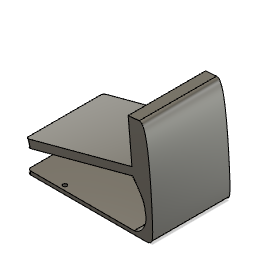
Iron_ Board Clip V2 (Autodesk Fusion 360 design; units mm, degrees)
Autodesk Fusion 360 part; units mm, degrees
sketch "Pi Plate" plane through (0, 0, 0) normal (0, 1, 0) x (1, 0, 0)
  line L0 (0, 0) -> (0, -56)
  line L1 (0, 0) -> (85, 0)
  line L2 (85, 0) -> (85, -56)
  line L3 (85, -56) -> (0, -56)
  line L4 (81.5, 0) -> (81.5, -3.5) construction
  line L5 (81.5, -3.5) -> (85, -3.5) construction
  circle A0 centre (81.5, -3.5) radius 1.425
  line L6 (0, -28) -> (85, -28) construction
  circle A1 centre (81.5, -52.5) radius 1.425
  line L7 (81.5, -3.5) -> (23.5, -3.5) construction
  circle A2 centre (23.5, -3.5) radius 1.425
  circle A3 centre (23.5, -52.5) radius 1.425
  line L8 (85, 0) -> (85, -15)
  line L9 (85, -15) -> (93, -15)
  line L10 (93, -15) -> (93, -5)
  line L11 (93, -5) -> (85, -5)
  dimension "d1" = 56
  dimension "d2" = 85
  dimension "d3" = 3.5
  dimension "d4" = 3.5
  dimension "d6" = 2.85
  dimension "d7" = 58
  dimension "d8" = 2.85
  dimension "d37" = 15
  dimension "d38" = 8
  dimension "d39" = 10
  constraint coincident L0.start L1.start
  constraint vertical L0
  constraint perpendicular L0 L1
  constraint perpendicular L1 L2
  constraint perpendicular L2 L3
  constraint coincident L1 L4.start
  constraint perpendicular L1 L4
  constraint coincident L2 L5.end
  constraint perpendicular L2 L5
  constraint coincident L4.end L5.start
  constraint midpoint L0 L6.start
  constraint midpoint L2 L6.end
  constraint symmetric A0 L6 A1
  constraint perpendicular L4 L7
  constraint coincident L7.end A2.centre
  constraint symmetric L6 A2 A3
  constraint perpendicular L5 L8
  constraint perpendicular L8 L9
  constraint perpendicular L9 L10
  constraint coincident L2 L11.end
  measures "d1" distance of L0.start L0.end
  measures "d2" distance of L0.start L1.end
  measures "d3" distance of L4.start L4.end
  measures "d4" distance of L4.end L5.end
  measures "d6" diameter of A0
  measures "d7" distance of L4.end L7.end
  measures "d8" diameter of A2
  measures "d37" distance of L1.end L8.end
  measures "d38" distance of L8.end L9.end
  measures "d39" distance of L9.end L10.end
extrude "Extrude1" add sketch "Pi Plate" along normal blind 2.5 contours L0 L1 L2 L3 L8
sketch "Clip Side" plane through (0, 0, 56) normal (0, 0, 1) x (1, 0, 0)
  line L0 (0, 0) -> (85, 0)
  line L1 (85, 0) -> (85, 2.5)
  line L2 (85, 2.5) -> (0, 2.5)
  line L3 (0, 2.5) -> (0, 0)
  line L4 (85, 2.5) -> (75.9413, 36.3074) construction
  line L5 (85, 2.5) -> (90, 2.5153)
  line L6 (0, 2.5) -> (0, 15.959)
  line L7 (0, 15.959) -> (75.9413, 36.3074)
  line L8 (74.5178, 41.62) -> (-1.4235, 21.2716)
  line L9 (-1.4235, 21.2716) -> (0, 15.959)
  line L10 (80.4707, 19.4037) -> (138.9269, 35.067) construction
  line L11 (75.9413, 36.3074) -> (84.1517, 38.5074)
  line L12 (72.7687, 72.5706) -> (80.7383, 73.2679)
  line L13 (80.7383, 73.2679) -> (84.1517, 38.5074)
  spline S0 degree 5 poles (85, 0) (85.7038, -0.0126) (86.9919, 0.0407) (88.5662, 0.3597) (89.9346, 1.2401) (90.5461, 4.0966) (90.5133, 11.1599) (90.0253, 22.2132) (89.1744, 36.0508) (87.9366, 50.5661) (86.2276, 63.3649) (84.3878, 70.3523) (82.6924, 72.9385) (81.4143, 73.373) (80.7383, 73.2679) knots 0 0 0 0 0 0 0.1 0.2 0.3 0.4 0.5 0.6 0.7 0.8 0.9 1 1 1 1 1 1
  line L14 (82.5373, 73.5477) -> (78.9392, 72.988)
  line L15 (89.2071, -0.1554) -> (90.7928, 5.1861)
  line L16 (75.9413, 36.3074) -> (72.7687, 72.5706)
  line L17 (74.5178, 41.62) -> (75.9413, 36.3074)
  spline S1 degree 5 poles (77.0666, 2.5) (77.518, 2.582) (78.4018, 2.8013) (79.6705, 3.2963) (81.246, 4.2904) (82.9988, 6.0816) (84.4519, 8.3641) (85.4854, 11.012) (85.8037, 13.7661) (85.5761, 16.347) (85.1435, 18.5645) (84.827, 20.3572) (84.5732, 21.9602) (83.9831, 23.7933) (82.9151, 26.0418) (81.2588, 28.8315) (79.4414, 31.5279) (77.799, 33.8154) (76.5811, 35.4573) (75.9413, 36.3074) knots 0 0 0 0 0 0 0.066667 0.133333 0.2 0.266667 0.333333 0.4 0.466667 0.533333 0.6 0.666667 0.733333 0.8 0.866667 0.933333 1 1 1 1 1 1
  line L18 (85.1921, 18.349) -> (84.3983, 22.7759)
  line L19 (74.5178, 41.62) -> (75.4546, 41.871)
  line L20 (74.355, 54.439) -> (84.8151, 55.3541) construction
  line L21 (83.6776, 68.3559) -> (85.9526, 42.3523) construction
  line L22 (83.6443, 6.1062) -> (86.3557, 13.8938)
  point P0 (84.7952, 20.5625)
  point P1 (85, 10)
  dimension "d12" = 35
  dimension "d13" = 5
  dimension "d15" = 5.5
  dimension "d16" = 31
  dimension "d18" = 8.5
  dimension "d36" = 75
  dimension "d50" = 10.5
  dimension "d51" = 8
  dimension "d52" = 14.8786
  dimension "d53" = 80
  constraint coincident L1.end L2.start
  constraint perpendicular L2 L6
  constraint perpendicular L4 L7
  constraint perpendicular L7 L9
  constraint midpoint L4 L10.start
  constraint perpendicular L4 L10
  constraint perpendicular L4 L11
  constraint coincident L0.end L1.start
  constraint midpoint L12.end L14
  constraint midpoint L5.end L15
  constraint perpendicular L11 L17
  constraint perpendicular L8 L9
  constraint coincident L10 P0
  constraint midpoint P0 L18
  constraint coincident L16 L19.end
  constraint parallel L8 L19
  constraint perpendicular L12 L16
  constraint coincident L2 L1.end
  constraint coincident L2 S1.start
  constraint midpoint L16 L20.start
  constraint perpendicular L16 L20
  constraint midpoint L20.end L21
  constraint perpendicular L20 L21
  constraint coincident L2.end L3.start
  constraint midpoint P1 L22
  measures "d12" distance of L1.end L4.end
  measures "d13" distance of L1.end L5.end
  measures "d15" distance of L4.end L8.start
  measures "d16" distance of L8.start L12.start
  measures "d18" distance of L4.end L11.end
  measures "d36" angle of L2 L4
  measures "d50" distance of L20.start L20.end
  measures "d51" distance of L12.end L16
  measures "d53" angle of L7 L16
extrude "Extrude2" add sketch "Clip Side" against normal up to surface (56 mm away) contours L1 L5 S0 | L2 L5 L11 L13 S0 S1 | L7 L8 L9 L17 | L11 L12 L13 L16 | L16 L17 L19
sketch "Sensor Plate" plane through (78.5168, 6.8693, 0) normal (-0.996195, -0.087156, 0) x (0, 0, 1)
  line L0 (28.3175, 79.196) -> (28.3175, 50.0437) construction
  line L1 (56, 50.5438) -> (0, 50.5438) construction
  line L2 (28.3175, 63.8938) -> (14.9675, 63.8938)
  line L3 (14.9675, 63.8938) -> (14.9675, 50.5438)
  line L4 (28.3175, 63.8938) -> (41.6675, 63.8938)
  line L5 (41.6675, 63.8938) -> (41.6675, 50.5438)
  line L6 (14.9675, 37.1938) -> (14.9675, 50.5438)
  line L7 (28.3175, 37.1938) -> (14.9675, 37.1938)
  line L8 (28.3175, 37.1938) -> (41.6675, 37.1938)
  line L9 (41.6675, 37.1938) -> (41.6675, 50.5438)
  line L10 (17.8575, 63.8938) -> (17.8575, 61.0038) construction
  line L11 (17.8575, 61.0038) -> (14.9675, 61.0038) construction
  circle A0 centre (17.8575, 61.0038) radius 1.425
  circle A1 centre (38.7775, 61.0038) radius 1.425
  circle A2 centre (38.7775, 40.0838) radius 1.425
  circle A3 centre (17.8575, 40.0838) radius 1.425
  line L12 (14.9675, 37.1938) -> (22.9675, 37.1938)
  line L13 (41.6675, 37.1938) -> (33.6675, 37.1938)
  line L14 (0, 5.5) -> (56, 5.5)
  line L15 (56, 5.5) -> (56, 40.5)
  line L16 (0, 40.5) -> (0, 5.5)
  line L17 (0, 23) -> (56, 23) construction
  line L18 (0, 0) -> (15, 0)
  line L19 (33.6675, 37.1938) -> (15, 0)
  line L20 (0, 0) -> (5, 0)
  line L21 (22.9675, 37.1938) -> (5, 0)
  line L22 (0, 65.9522) -> (0, 35.1354)
  line L23 (56, 35.1354) -> (56, 65.9522)
  line L24 (56, 65.9522) -> (0, 65.9522)
  line L25 (0, 35.1354) -> (56, 35.1354)
  line L26 (56, -4.2263) -> (0, -4.2263)
  line L27 (22.9675, 37.1938) -> (28.3175, 37.1938)
  dimension "d21" = 13.35
  dimension "d22" = 13.35
  dimension "d24" = 2.89
  dimension "d25" = 2.85
  dimension "d26" = 8
  dimension "d27" = 15
  dimension "d32" = 5
  constraint coincident L0 L2.start
  constraint perpendicular L0 L2
  constraint coincident L1 L3.end
  constraint perpendicular L1 L3
  constraint symmetric L0 L2.start L4.start
  constraint symmetric L0 L2.end L4.end
  constraint symmetric L0 L3.end L5.end
  constraint symmetric L1 L2.start L7.start
  constraint symmetric L1 L2.end L6.start
  constraint symmetric L1 L3.end L6.end
  constraint symmetric L1 L4.end L8.end
  constraint symmetric L1 L5.end L9.end
  constraint coincident L3 L11.end
  constraint perpendicular L3 L11
  constraint equal L10 L11
  constraint perpendicular L10 L11
  constraint coincident L2 L10.start
  constraint coincident L10.end L11.start
  constraint symmetric L0 A0 A1
  constraint symmetric L1 A0 A3
  constraint symmetric L1 A1 A2
  constraint perpendicular L6 L12
  constraint symmetric L0 L6.start L8.end
  constraint symmetric L0 L12.end L13.end
  constraint midpoint L16 L17.start
  constraint midpoint L15 L17.end
  constraint coincident L18.start L20.start
  constraint perpendicular L16 L18
  constraint coincident L18 L20.end
  constraint coincident L1.end L22
  constraint coincident L1 L5.end
  constraint horizontal L1
  constraint midpoint L1.start L23
  measures "d21" distance of L2.start L2.end
  measures "d22" distance of L2.end L3.end
  measures "d24" distance of L10.end L11.end
  measures "d25" diameter of A0
  measures "d26" distance of L6.start L12.end
  measures "d27" distance of L18.start L18.end
  measures "d32" distance of L18.start L20.end
extrude "Extrude3" cut sketch "Sensor Plate" against normal blind 6.5 contours L2 L3 L4 L5 L6 L7 L8 L9 L12 L13 L27 | L7 L8 L19 L21 L25 L27 | L14 L19 L21 L25 | L14 L18 L19 L21
extrude "Extrude6" [suppressed]
extrude "Extrude4" cut sketch "Sensor Plate" against normal blind 10.5 contours A0 | A1 | A2 | A3
extrude "Extrude5" [suppressed]
fillet "Fillet2" radius 2 4 edges at (-0.7118, 18.6153, 0) (-0.7118, 18.6153, 56) (0, 1.25, 56) (0, 1.25, 0)
equation "d4 = d3"
equation "m3_screw_hole = 2.85 mm"
equation "d6 = m3_screw_hole"
equation "d8 = m3_screw_hole"
equation "screw_depth = 5.5 mm"
equation "d10 = screw_depth - wall_thickness"
equation "wall_thickness = 3 mm"
equation "d15 = screw_depth"
equation "d16 = 28 mm + wall_thickness"
equation "hole_tolerance = 0.7 mm"
equation "d18 = screw_depth + wall_thickness"
equation "d21 = 13 mm + ( hole_tolerance * 0.5 )"
equation "d22 = d21"
equation "d24 = 2.54 mm + ( hole_tolerance / 2 )"
equation "d25 = m3_screw_hole"
equation "d30 = -5 mm - screw_depth"
equation "d40 = screw_depth + 8 mm"
equation "d50 = 5 mm + screw_depth"
equation "d51 = 5 mm + wall_thickness"
